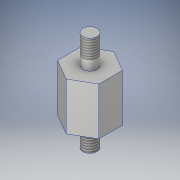
# Autodesk Inventor part: spacer
Saved by Autodesk Inventor 2018 (Build 220112000, 112)
## iProperties
Created: 2021-04-18
Part Number: spacer
Material: Aluminum 6061
Document SubType Name: Modeling
Designer: Ramana Bharathi
Density: 2.7 g/cm^3
Appearance: Aluminum - Flat
Mass: 1.96364 g
Surface Area: 5.33576 cm^2
Volume: 0.727273 cm^3
Author: Ramana Bharathi
Autodesk Inventor part; units mm, degrees
ref_plane "YZ Plane" through (0, 0, 0) normal (1, 0, 0) x (0, 1, 0)
ref_plane "XZ Plane" through (0, 0, 0) normal (0, 1, 0) x (-1, 0, 0)
ref_plane "XY Plane" through (0, 0, 0) normal (0, 0, 1) x (1, 0, 0)
sketch "Sketch1" plane through (0, 0, 0) normal (0, 1, 0) x (-1, 0, 0)
  line L0 (0, -5) -> (-4.3301, -2.5)
  line L1 (-4.3301, -2.5) -> (-4.3301, 2.5)
  line L2 (-4.3301, 2.5) -> (0, 5)
  line L3 (0, 5) -> (4.3301, 2.5)
  line L4 (4.3301, 2.5) -> (4.3301, -2.5)
  line L5 (4.3301, -2.5) -> (0, -5)
  point P0 (0, 0)
  point P1 (0, 0)
  point P2 (0, 0)
  dimension "d1" = 5
  constraints: 12 end point, 2 coincident, 13 other
  measures "d1" distance of L0.end L1.end
extrude "Extrusion1" add sketch "Sketch1" along normal blind 10
sketch "Sketch2" plane through (0, 10, 0) normal (0, 1, 0) x (1, 0, 0)
  circle A0 centre (0, 0) radius 1.5
  dimension "d4" = 3
  constraints: 1 centre point, 1 coincident
  measures "d4" diameter of A0
extrude "Extrusion2" add sketch "Sketch2" along normal blind 6
sketch "Sketch3" plane through (0, 0, 0) normal (0, -1, 0) x (1, 0, 0)
  circle A0 centre (0, 0) radius 1.5
  dimension "d7" = 3
  constraints: 1 centre point, 1 coincident
  measures "d7" diameter of A0
extrude "Extrusion3" add sketch "Sketch3" along normal blind 5
thread "Thread1" size "M3x0.5" class "6g" standard "ANSI Metric M Profile" length 4
thread "Thread2" size "M3x0.5" class "6g" standard "ANSI Metric M Profile" full length
body "Solid1"
